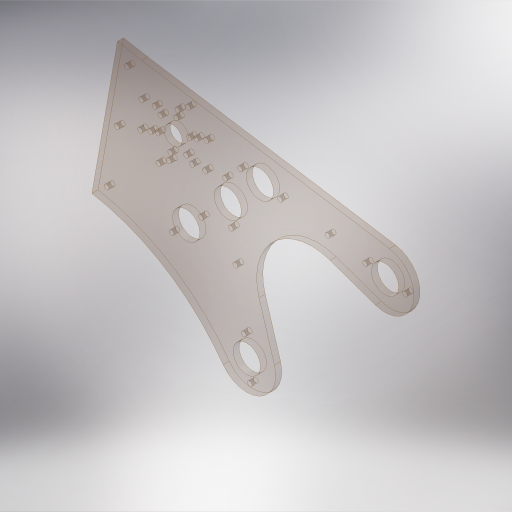
# Autodesk Inventor part: GP7-001
Saved by Autodesk Inventor 2023.4 (Build 274418000, 418)
## iProperties
Created: 2025-02-24
Part Number: GP7-001
Material: Polycarbonate, Smoke
Document SubType Name: Modeling
Designer: dlangdon
Density: 1.2 g/cm^3
Appearance: Polycarbonate - Smoked
Author: dlangdon
Autodesk Inventor part; units mm, degrees
ref_plane "YZ Plane" through (0, 0, 0) normal (1, 0, 0) x (0, 1, 0)
ref_plane "XZ Plane" through (0, 0, 0) normal (0, 1, 0) x (-1, 0, 0)
ref_plane "XY Plane" through (0, 0, 0) normal (0, 0, 1) x (1, 0, 0)
sketch "Sketch1" plane through (0, 0, 0) normal (0, 0, 1) x (1, 0, 0)
  circle A0 centre (71.842, 71.842) radius 50.8 construction
  circle A1 centre (-71.842, -71.842) radius 50.8 construction
  circle A2 centre (0, 0) radius 50.8 construction
  line L0 (-35.921, -35.921) -> (35.921, 35.921) construction
  line L1 (71.842, 71.842) -> (-71.842, -71.842) construction
  line L2 (-4.3707, 6.2419) -> (-4.3707, 50.6116) construction
  line L3 (-226.8798, -122.642) -> (638.5123, -122.642) construction
  circle A3 centre (147.8406, -65.492) radius 57.15 construction
  circle A4 centre (71.842, 71.842) radius 14.2621
  circle A5 centre (-71.842, -71.842) radius 14.2621
  circle A6 centre (-4.3707, 6.2419) radius 57.15 construction
  circle A7 centre (-71.842, -71.842) radius 30.1371 construction
  circle A8 centre (71.842, 71.842) radius 30.1371 construction
  circle A9 centre (-58.1561, 92.2961) radius 14.2621
  line L4 (-58.1561, 92.2961) -> (71.842, 71.842) construction
  circle A10 centre (71.842, 71.842) radius 14.3256 construction
  circle A11 centre (-71.842, -71.842) radius 14.3256 construction
  circle A12 centre (-91.5361, 58.2734) radius 14.2621
  line L5 (-71.842, -71.842) -> (-91.5361, 58.2734) construction
  circle A13 centre (-91.5361, 58.2734) radius 23.8316 construction
  circle A14 centre (-58.1561, 92.2961) radius 23.8316 construction
  line L6 (14.7165, 60.1103) -> (61.7767, 43.4355)
  line L7 (-43.0113, -63.0652) -> (-59.0434, -10.4018)
  arc A15 (14.7165, 60.1103) -> (-59.0434, -10.4018) centre (-4.3707, 6.2419) ccw
  line L8 (-206.2644, 146.6716) -> (-181.2503, 142.2609)
  line L9 (-181.2503, 142.2609) -> (-207.7142, -7.8238) construction
  line L10 (-207.7142, -7.8238) -> (-232.7284, -3.4132) construction
  line L11 (-232.7284, -3.4132) -> (-206.2644, 146.6716) construction
  line L12 (-248.4004, -92.2937) -> (35.0702, -142.2772) construction
  line L13 (-201.8537, 171.6857) -> (174.1389, 105.388) construction
  line L14 (-201.8537, 171.6857) -> (-248.4004, -92.2937) construction
  circle A16 centre (-148.3902, 90.9262) radius 31.75 construction
  line L15 (-87.9696, 34.7102) -> (-79.4445, -21.6141) construction
  circle A17 centre (12.2502, 81.2183) radius 9.525 construction
  line L16 (-193.7573, 144.4662) -> (-220.2213, -5.6185) construction
  line L17 (-196.514, 128.8324) -> (-217.4646, 10.0153) construction
  circle A18 centre (-148.3902, 90.9262) radius 17.4625 construction
  circle A19 centre (-148.3902, 90.9262) radius 9.525
  circle A20 centre (-58.1561, 92.2961) radius 30.1816 construction
  line L18 (-206.2644, 146.6716) -> (-232.7284, -3.4132)
  arc A21 (61.7767, 43.4355) -> (76.5363, 101.6113) centre (71.842, 71.842) ccw
  arc A22 (-96.3608, -89.3657) -> (-43.0113, -63.0652) centre (-71.842, -71.842) ccw
  line L19 (-148.3902, 90.9262) -> (-131.9808, 96.8987) construction
  line L20 (-114.0797, 103.4142) -> (-182.7007, 78.4382) construction
  circle A23 centre (-182.7007, 78.4382) radius 4.7625 construction
  line L21 (0, 0) -> (-4.3707, 6.2419) construction
  circle A24 centre (71.842, 71.842) radius 28.6512 construction
  line L22 (64.3208, 44.1957) -> (-61.9, 78.5341) construction
  line L23 (73.1739, 100.4623) -> (-57.4931, 106.5427) construction
  line L24 (-181.2503, 142.2609) -> (76.5363, 101.6113)
  line L25 (-148.3902, 90.9262) -> (-134.757, 17.1048) construction
  circle A25 centre (-134.757, 17.1048) radius 31.75 construction
  circle A26 centre (-134.757, 17.1048) radius 14.2621
  line L26 (-91.5361, 58.2734) -> (-134.757, 17.1048) construction
  circle A27 centre (-148.3902, 90.9262) radius 25.4 construction
  arc A28 (-96.3608, -89.3657) -> (-232.7284, -3.4132) centre (-269.7327, -213.2752) ccw
  circle A29 centre (-148.3902, 90.9262) radius 36.5125 construction
  line L27 (-181.4818, 106.357) -> (-148.3902, 90.9262) construction
  point P0 (-83.707, 6.548)
  point P1 (-206.9893, 69.4239)
  point P2 (-206.9893, 69.4239)
  point P3 (-145.3579, 108.1234)
  point P4 (-161.7673, 102.1508)
  point P5 (-164.7996, 84.9536)
  point P6 (-151.4225, 73.729)
  point P7 (-135.0132, 79.7015)
  point P8 (-124.522, 99.6135)
  point P9 (-143.9796, 115.9403)
  point P10 (-167.8477, 107.253)
  point P11 (-172.2584, 82.2388)
  point P12 (-152.8009, 65.912)
  point P13 (-128.9327, 74.5994)
  point P14 (-160.8782, 125.2367)
  point P15 (-135.9022, 56.6156)
  point P16 (-132.9594, 124.0177)
  point P17 (-163.8211, 57.8346)
  point P18 (-115.2987, 75.4953)
  dimension "d7" = 101.6
  dimension "d18" = 47.6631
  dimension "d34" = 34.925
  dimension "d65" = 50.8
  dimension "d3" = 45
  dimension "d4" = 0
  dimension "d8" = 101.6
  dimension "d9" = 28.5242
  dimension "d10" = 101.6
  dimension "d11" = 114.3
  dimension "d12" = 114.3
  dimension "d13" = 15.875
  dimension "d14" = 15.875
  dimension "d15" = 131.5974
  dimension "d16" = 28.6512
  dimension "d17" = 131.5974
  dimension "d19" = 47.6631
  dimension "d22" = 25.4
  dimension "d23" = 152.4
  dimension "d26" = 268.0517
  dimension "d27" = 63.5
  dimension "d30" = 203.2
  dimension "d31" = 10
  dimension "d32" = 19.05
  dimension "d33" = 120.65
  dimension "d35" = 19.05
  dimension "d36" = 6.35
  dimension "d40" = 360
  dimension "d44" = 9.525
  dimension "d55" = 80
  dimension "d56" = 7.62
  dimension "d57" = 25.4
  dimension "d58" = 57.3024
  dimension "d59" = 63.5
  dimension "d60" = 75.0697
  dimension "d61" = 59.69
  dimension "d62" = 55
  dimension "d68" = 360
  dimension "d70" = 41.275
  dimension "d71" = 60
  dimension "d82" = 360
  dimension "d87" = 360
  dimension "d89" = 45
  constraints: 56 end point, 26 centre point, 24 coincident, 23 point on circle, 16 tangent, 7 midpoint, 6 equal radius, 5 point on line, 4 collinear, 4 parallel, 2 horizontal, 1 concentric, 1 perpendicular, 1 vertical, 39 other
  measures "d3" angle of L2 L0
  measures "d4" distance between parallel lines of L0 L1
  measures "d8" diameter of A2
  measures "d9" diameter of A4
  measures "d10" diameter of A0
  measures "d11" diameter of A3
  measures "d12" diameter of A6
  measures "d13" radial gap between concentric circles of A5 A7
  measures "d14" radial gap between concentric circles of A4 A8
  measures "d15" distance of L4.start L4.end
  measures "d16" diameter of A10
  measures "d17" distance of L5.start L5.end
  measures "d19" diameter of A14
  measures "d22" distance of L9.end L10.end
  measures "d23" distance of L10.end L8.start
  measures "d26" distance of L13.start L12.start
  measures "d27" diameter of A16
  measures "d30" distance from line of point (0, 0) L9
  measures "d31" angle of L3 L12
  measures "d32" diameter of A17
  measures "d33" distance of L17.start L17.end
  measures "d35" diameter of A19
  measures "d36" radial gap between concentric circles of A14 A20
  measures "d44" diameter of A23
  measures "d55" angle of L1 L21
  measures "d56" distance of L21.start L21.end
  measures "d57" distance between parallel lines of L13 L8
  measures "d58" diameter of A24
  measures "d59" diameter of A25
  measures "d60" distance of L19.start L25.end
  measures "d61" distance of L26.start L26.end
  measures "d62" angle of L15 L26
  measures "d70" distance from line of L9 L19.start
  measures "d71" angle of L9 L20
  measures "d89" angle of L20 L27
extrude "Extrusion1" add sketch "Sketch1" along normal blind 6.35
hole "Hole1" at (12.2502, 81.2183, 0) at (-196.514, 128.8324, 0) at (-206.9893, 69.4239, 0) at (-217.4646, 10.0153, 0) at (-131.9808, 96.8987, 0) at (-145.3579, 108.1234, 0) at (-161.7673, 102.1508, 0) at (-164.7996, 84.9536, 0) at (-151.4225, 73.729, 0) at (-135.0132, 79.7015, 0) at (-114.0797, 103.4142, 0) at (-182.7007, 78.4382, 0) at (-152.8009, 65.912, 0) at (-172.2584, 82.2388, 0) at (-167.8477, 107.253, 0) at (-143.9796, 115.9403, 0) at (-124.522, 99.6135, 0) at (-128.9327, 74.5994, 0) at (-83.707, 6.548, 0) at (-181.4818, 106.357, 0) at (-132.9594, 124.0177, 0) at (-115.2987, 75.4953, 0) at (-163.8211, 57.8346, 0) direction (0, 0, 1) diameter 5.1054 end through all clearance for "Flat Head Machine Screw (82)" size "#10" standard "Ansi Unified Screw Threads"
sketch "Sketch2" plane through (0, 0, 6.35) normal (0, 0, 1) x (1, 0, 0)
  circle A0 centre (-128.9327, 74.5994) radius 2.5527 construction
  circle A1 centre (-143.9796, 115.9403) radius 2.5527 construction
  circle A2 centre (-172.2584, 82.2388) radius 2.5527 construction
  circle A3 centre (-182.7007, 78.4382) radius 2.5527 construction
  circle A4 centre (-135.0132, 79.7015) radius 2.5527 construction
  circle A5 centre (-164.7996, 84.9536) radius 2.5527 construction
  circle A6 centre (-145.3579, 108.1234) radius 2.5527 construction
  circle A7 centre (-217.4646, 10.0153) radius 2.5527 construction
  circle A8 centre (-196.514, 128.8324) radius 2.5527 construction
  circle A9 centre (12.2502, 81.2183) radius 2.5527 construction
  circle A10 centre (-206.9893, 69.4239) radius 2.5527 construction
  circle A11 centre (-131.9808, 96.8987) radius 2.5527 construction
  circle A12 centre (-161.7673, 102.1508) radius 2.5527 construction
  circle A13 centre (-151.4225, 73.729) radius 2.5527 construction
  circle A14 centre (-114.0797, 103.4142) radius 2.5527 construction
  circle A15 centre (-152.8009, 65.912) radius 2.5527 construction
  circle A16 centre (-167.8477, 107.253) radius 2.5527 construction
  circle A17 centre (-124.522, 99.6135) radius 2.5527 construction
  circle A18 centre (-83.707, 6.548) radius 2.5527 construction
  line L0 (-43.0113, -63.0652) -> (-59.0434, -10.4018) construction
  arc A19 (14.7165, 60.1103) -> (-59.0434, -10.4018) centre (-4.3707, 6.2419) ccw construction
  line L1 (14.7165, 60.1103) -> (61.7767, 43.4355) construction
  arc A20 (61.7767, 43.4355) -> (76.5363, 101.6113) centre (71.842, 71.842) ccw construction
  line L2 (76.5363, 101.6113) -> (-181.2503, 142.2609) construction
  line L3 (-181.2503, 142.2609) -> (-206.2644, 146.6716) construction
  line L4 (-206.2644, 146.6716) -> (-232.7284, -3.4132) construction
  arc A21 (-96.3608, -89.3657) -> (-232.7284, -3.4132) centre (-269.7327, -213.2752) ccw construction
  arc A22 (-96.3608, -89.3657) -> (-43.0113, -63.0652) centre (-71.842, -71.842) ccw construction
  circle A23 centre (-91.5361, 58.2734) radius 14.2621 construction
  circle A24 centre (-148.3902, 90.9262) radius 9.525 construction
  circle A25 centre (-134.757, 17.1048) radius 14.2621 construction
  circle A26 centre (-58.1561, 92.2961) radius 14.2621 construction
  circle A27 centre (-71.842, -71.842) radius 14.2621 construction
  circle A28 centre (71.842, 71.842) radius 14.2621 construction
  line L5 (-74.9875, -51.0602) -> (-68.6965, -92.6238) construction
  line L6 (-149.9763, 2.6082) -> (-119.5377, 31.6014) construction
  line L7 (-94.6816, 79.0552) -> (-88.3906, 37.4916) construction
  line L8 (-78.9191, 95.5629) -> (-37.393, 89.0292) construction
  line L9 (51.079, 75.1089) -> (92.6051, 68.5752) construction
  circle A29 centre (-91.5361, 58.2734) radius 14.2621 construction
  line L10 (-58.1561, 92.2961) -> (-91.5361, 58.2734) construction
  line L11 (-58.1561, 92.2961) -> (71.842, 71.842) construction
  line L12 (-91.5361, 58.2734) -> (-134.757, 17.1048) construction
  line L13 (-91.5361, 58.2734) -> (-71.842, -71.842) construction
  point P0 (0, 0)
  dimension "d72" = 42.037
  constraints: 19 end point, 14 coincident, 5 collinear, 5 midpoint, 4 equal length
  measures "d72" distance of L5.start L5.end
hole "Hole2" at (-74.9875, -51.0602, 6.35) at (-119.5377, 31.6014, 6.35) at (-68.6965, -92.6238, 6.35) at (-149.9763, 2.6082, 6.35) at (-88.3906, 37.4916, 6.35) at (-94.6816, 79.0552, 6.35) at (-37.393, 89.0292, 6.35) at (-78.9191, 95.5629, 6.35) at (92.6051, 68.5752, 6.35) at (51.079, 75.1089, 6.35) direction (0, 0, -1) diameter 5.1054 end through all clearance for "Flat Head Machine Screw (82)" size "#10" standard "Ansi Unified Screw Threads"
body "Solid1"
